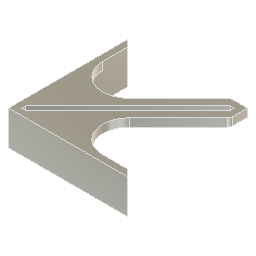
Нахождение центра без краев (Autodesk Fusion 360 design; units mm, degrees)
Autodesk Fusion 360 part; units mm, degrees
sketch "Sketch1" plane through (0, 0, 0) normal (0, 0, 1) x (1, 0, 0)
  line L0 (-22.5, 22.5) -> (-22.5, -22.5)
  line L1 (-22.5, -22.5) -> (22.5, -22.5)
  line L2 (22.5, 16.9645) -> (22.5, 22.5)
  line L3 (-20, 20) -> (-20, 10.5061)
  line L4 (20, 20) -> (18.5858, 20)
  line L5 (-20, 20) -> (-22.5, 22.5)
  line L6 (-2.9289, 3.435) -> (15.5503, 21.9142)
  line L7 (22.5, 22.5) -> (16.9645, 22.5)
  line L8 (10.5061, -20) -> (20, -20)
  line L9 (20, -20) -> (22.5, -22.5)
  line L10 (3.435, -2.9289) -> (21.9142, 15.5503)
  line L11 (20, 18.5858) -> (20, 20)
  arc A0 (3.435, -2.9289) -> (10.5061, -20) centre (10.5061, -10) ccw
  arc A1 (-20, 10.5061) -> (-2.9289, 3.435) centre (-10, 10.5061) ccw
  line L12 (-18.5858, -20) -> (-20, -20)
  line L13 (-20, -18.5858) -> (-20, -20)
  line L14 (-18.5858, -20) -> (20, 18.5858)
  line L15 (-20, -18.5858) -> (18.5858, 20)
  arc A2 (21.9142, 15.5503) -> (22.5, 16.9645) centre (20.5, 16.9645) ccw
  arc A3 (16.9645, 22.5) -> (15.5503, 21.9142) centre (16.9645, 20.5) ccw
  line L16 (-20, 20) -> (-20, -18.5858)
  line L17 (20, -20) -> (-18.5858, -20)
  dimension "d3" = 45
  dimension "d4" = 45
  dimension "d5" = 10
  dimension "d6" = 2
  constraint horizontal L8
  constraint perpendicular L8 L11
  constraint parallel L4 L8
  constraint parallel L3 L11
  constraint horizontal L1
  constraint perpendicular L1 L2
  constraint parallel L1 L7
  constraint parallel L0 L2
  constraint parallel L5 L9
  constraint coincident L8 L12.start
  constraint coincident L3 L13.start
  constraint tangent L10 A0
  constraint tangent L8 A0
  constraint tangent L6 A1
  constraint tangent L3 A1
  constraint equal A0 A1
  constraint horizontal L12
  constraint perpendicular L12 L13
  constraint tangent L2 A2
  constraint tangent L10 A2
  constraint tangent L7 A3
  constraint tangent L6 A3
  constraint equal A2 A3
  measures "d3" distance of L2.end L0.start
  measures "d4" distance of L2.end L1.end
  measures "d5" radius of A0
  measures "d6" radius of A2
extrude "Extrude1" add sketch "Sketch1" along normal blind 3 contours L0 L1 L3 L5 L8 L9 L12 L13 L16 L17 | L2 L4 L6 L7 L10 L11 A0 A1 L14 L15 A2 A3 L16 L17
extrude "Extrude2" add sketch "Sketch1" against normal blind 10 contours L0 L1 L3 L5 L8 L9 L12 L13 L16 L17
